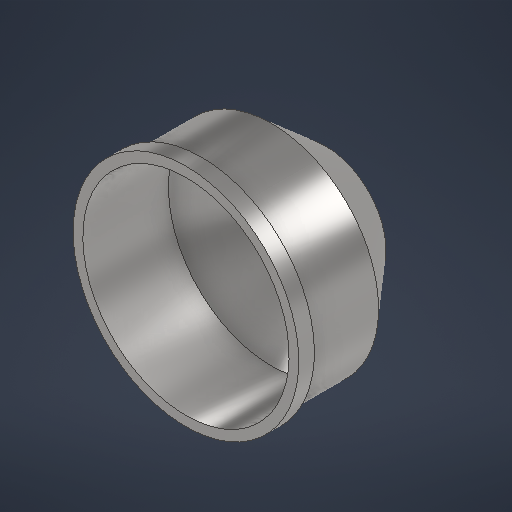
# Autodesk Inventor part: DiscoCorpoScarico
Saved by Autodesk Inventor 2026.2 (Build 302298010, 298A)
## iProperties
Created: 2026-04-30
Part Number: DiscoCorpoScarico
Material: Steel, Alloy
Document SubType Name: Modeling
Designer: Yan
Density: 7.73 g/cm^3
Appearance: Semi-Polished
Author: Yan
Autodesk Inventor part; units mm, degrees
ref_plane "YZ Plane" through (0, 0, 0) normal (1, 0, 0) x (0, 1, 0)
ref_plane "XZ Plane" through (0, 0, 0) normal (0, 1, 0) x (-1, 0, 0)
ref_plane "XY Plane" through (0, 0, 0) normal (0, 0, 1) x (1, 0, 0)
sketch "Sketch1" plane through (0, 0, 0) normal (1, 0, 0) x (0, 1, 0)
  line L0 (0, 0) -> (0, -360)
  line L1 (0, 0) -> (3.9526, 0)
  line L2 (3.9526, 0) -> (290, 0)
  line L3 (290, 0) -> (290, -40)
  line L4 (290, -40) -> (275, -40)
  line L5 (275, -40) -> (275, -220)
  line L6 (140, -360) -> (0, -360)
  line L7 (265, -220) -> (265, 0)
  line L8 (265, -220) -> (140, -360)
  line L9 (275, -220) -> (154, -360)
  line L10 (154, -360) -> (140, -360)
  dimension "d0" = 360
  dimension "d1" = 530
  dimension "d2" = 40
  dimension "d3" = 580
  dimension "d4" = 550
  dimension "d7" = 180
  dimension "d8" = 220
  dimension "d13" = 140
  dimension "d14" = 14
  constraints: 22 end point, 3 perpendicular, 2 horizontal, 2 point on line, 2 vertical
  measures "d0" distance of L0.start L0.end
  measures "d1" diameter of L7 L0
  measures "d2" distance between parallel lines of L4 L2
  measures "d3" diameter of L3 L0
  measures "d4" diameter of L5 L0
  measures "d7" distance of L4.end L5.end
  measures "d8" distance of L7.start L7.end
  measures "d13" distance of L6.start L0.end
  measures "d14" distance of L9.end L6.start
revolve "Revolution1" add sketch "Sketch1" angle 360 about axis through (0, 0, 0) along (0, 0, -1) contours L8 L7 L2 L3 L4 L5 L9 L10
body "Solid1"
